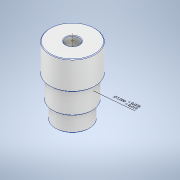
# Autodesk Inventor part: nabe
Saved by Autodesk Inventor 2022 (Build 260153000, 153)
## iProperties
Created: 2022-11-23
Part Number: nabe
Material: Aluminium 6061
Document SubType Name: Modeling
Designer: Friedrich Walmrath
Density: 2.7 g/cm^3
Appearance: Aluminium - flach
Author: Friedrich Walmrath
Autodesk Inventor part; units mm, degrees
ref_plane "YZ Plane" through (0, 0, 0) normal (1, 0, 0) x (0, 1, 0)
ref_plane "XZ Plane" through (0, 0, 0) normal (0, 1, 0) x (-1, 0, 0)
ref_plane "XY Plane" through (0, 0, 0) normal (0, 0, 1) x (1, 0, 0)
sketch "Skizze1" plane through (0, 0, 0) normal (0, 0, 1) x (1, 0, 0)
  line L0 (0, 5) -> (4, 5)
  line L1 (4, 5) -> (4, 0)
  line L2 (4, 0) -> (3, 0)
  line L3 (3, 0) -> (3, -7)
  line L4 (3, -7) -> (0, -7)
  line L5 (0, -7) -> (0, 5)
  line L6 (3.5, 0) -> (3.5, -4)
  line L7 (3.5, -4) -> (3, -4)
  point P0 (0, 0)
  dimension "d0" = 6
  dimension "d1" = 7
  dimension "d2" = 8
  dimension "d3" = 5
  dimension "d31" = 7
  dimension "d32" = 4
  constraints: 16 end point, 6 perpendicular, 2 point on line, 1 horizontal, 1 horizontal alignment, 1 midpoint, 1 vertical
  measures "d0" diameter of L3 L5
  measures "d1" distance of L2.end L3.end
  measures "d2" diameter of L1 L5
  measures "d3" distance of L0.end L1.end
  measures "d31" diameter of L6 L5
  measures "d32" distance of L6.start L6.end
revolve "Umdrehung1" add sketch "Skizze1" angle 360 about axis through (0, -7, 0) along (0, 1, 0)
chamfer "Fase1" distance 0.1 angle 45 4 edges at (-4, 5, 0) (-3, -7, 0) (-4, 0, 0) (-3.5, -4, 0)
hole "Bohrung1" at (0, 5, 0) direction (0, -1, 0) diameter 2.3 end through all both
chamfer "Fase2" distance 0.1 angle 45 2 edges at (0, -7, -1.15) (0, 5, -1.15)
sketch "Skizze2" plane through (0, 0, 0) normal (0, 0, 1) x (1, 0, 0)
  circle A0 centre (0, 2.5) radius 1
  line L0 (1.25, 5) -> (-1.25, 5) projected
  line L1 (0, 7.4) -> (0, -9.4) projected
  point P0 (0, 0)
  dimension "d20" = 2
  dimension "d21" = 2.5
  constraints: 1 centre point, 1 point on line
  measures "d20" diameter of A0
  measures "d21" distance from line of L0 A0.centre
extrude "Extrusion1" cut sketch "Skizze2" against normal blind 10
chamfer "Fase3" distance 0.1 angle 45 1 edges at (-1, 2.5012, -3.873)
thread "Gewinde1" size "M2x0.4" class "6H" standard "ANSI Metric M Profile" full length
